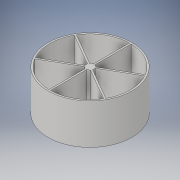
# Autodesk Inventor part: wheel
Saved by Autodesk Inventor 2019 (Build 230136000, 136)
## iProperties
Created: 2019-04-05
Part Number: wheel
Material: Generic
Document SubType Name: Modeling
Designer: jmc
Density: 1 g/cm^3
Appearance: Default
Author: jmc
Autodesk Inventor part; units mm, degrees
ref_plane "YZ Plane" through (0, 0, 0) normal (1, 0, 0) x (0, 1, 0)
ref_plane "XZ Plane" through (0, 0, 0) normal (0, 1, 0) x (-1, 0, 0)
ref_plane "XY Plane" through (0, 0, 0) normal (0, 0, 1) x (1, 0, 0)
sketch "Sketch1" plane through (0, 0, 0) normal (0, 1, 0) x (-1, 0, 0)
  line L0 (42.7926, 25.861) -> (42.8013, 25.866)
  line L1 (43.7926, 24.129) -> (43.8013, 24.134)
  line L2 (1, 50) -> (1, 49.99)
  line L3 (-1, 50) -> (-1, 49.99)
  line L4 (42.7926, -25.861) -> (42.8013, -25.866)
  line L5 (43.7926, -24.129) -> (43.8013, -24.134)
  line L6 (1, -49.99) -> (1, -50)
  line L7 (-1, -49.99) -> (-1, -50)
  line L8 (-42.8013, -25.866) -> (-42.7926, -25.861)
  line L9 (-43.8013, -24.134) -> (-43.7926, -24.129)
  line L10 (-43.8013, 24.134) -> (-43.7926, 24.129)
  line L11 (-42.8013, 25.866) -> (-42.7926, 25.861)
  line L12 (4.7426, 1.5835) -> (43.7926, 24.129)
  line L13 (4.7426, -1.5835) -> (43.7926, -24.129)
  line L14 (1, 49.99) -> (1, 4.899)
  line L15 (3.7426, 3.3155) -> (42.7926, 25.861)
  line L16 (-42.7926, 25.861) -> (-3.7426, 3.3155)
  line L17 (-1, 49.99) -> (-1, 4.899)
  line L18 (-43.7926, -24.129) -> (-4.7426, -1.5835)
  line L19 (-43.7926, 24.129) -> (-4.7426, 1.5835)
  line L20 (-42.7926, -25.861) -> (-3.7426, -3.3155)
  line L21 (-1, -4.899) -> (-1, -49.99)
  line L22 (3.7426, -3.3155) -> (42.7926, -25.861)
  line L23 (1, -4.899) -> (1, -49.99)
  circle A0 centre (0, 0) radius 52
  arc A1 (-1, 49.99) -> (-42.7926, 25.861) centre (0, 0) ccw
  arc A2 (-43.7926, 24.129) -> (-43.7926, -24.129) centre (0, 0) ccw
  arc A3 (-42.7926, -25.861) -> (-1, -49.99) centre (0, 0) ccw
  arc A4 (1, -49.99) -> (42.7926, -25.861) centre (0, 0) ccw
  arc A5 (43.7926, -24.129) -> (43.7926, 24.129) centre (0, 0) ccw
  arc A6 (42.7926, 25.861) -> (1, 49.99) centre (0, 0) ccw
  arc A7 (1, -4.899) -> (3.7426, -3.3155) centre (0, 0) ccw
  arc A8 (-3.7426, -3.3155) -> (-1, -4.899) centre (0, 0) ccw
  arc A9 (-4.7426, 1.5835) -> (-4.7426, -1.5835) centre (0, 0) ccw
  arc A10 (-1, 4.899) -> (-3.7426, 3.3155) centre (0, 0) ccw
  arc A11 (4.7426, -1.5835) -> (4.7426, 1.5835) centre (0, 0) ccw
  arc A12 (3.7426, 3.3155) -> (1, 4.899) centre (0, 0) ccw
  constraints: 48 end point, 24 point on circle, 13 centre point, 3 coincident
extrude "Extrusion1" add sketch "Sketch1" along normal blind 50
body "Solid1"
